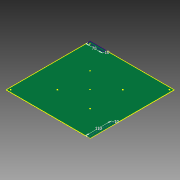
# Autodesk Inventor part: Platine
Saved by Autodesk Inventor 2013 SP1 (Build 170176100, 176)
## iProperties
Created: 2012-12-07
Part Number: Platine
Material: Platinengrün
Document SubType Name: Modeling
Designer: Sebastian
Density: 1 g/cm^3
Author: Sebastian
Autodesk Inventor part; units mm, degrees
ref_plane "YZ Plane" through (0, 0, 0) normal (1, 0, 0) x (0, 1, 0)
ref_plane "XZ Plane" through (0, 0, 0) normal (0, 1, 0) x (-1, 0, 0)
ref_plane "XY Plane" through (0, 0, 0) normal (0, 0, 1) x (1, 0, 0)
sketch "Skizze1" plane through (0, 0, 0) normal (0, 0, 1) x (1, 0, 0)
  line L0 (-180, -180) -> (180, -180)
  line L1 (180, -180) -> (180, 180)
  line L2 (180, 180) -> (-180, 180)
  line L3 (-180, 180) -> (-180, -180)
  line L4 (-180, -180) -> (180, 180) construction
  line L5 (180, -180) -> (-180, 180) construction
  point P0 (0, 0)
  dimension "d0" = 360
  dimension "d1" = 360
  constraints: 12 end point, 2 midpoint, 2 parallel, 1 horizontal, 1 perpendicular
  measures "d0" distance of L2.end L1.end
  measures "d1" distance of L1.end L0.end
extrude "Extrusion1" add sketch "Skizze1" along normal blind 2
hole "Bohrung1" at (-170, -170, 0) direction (0, 0, 1) diameter 3 end through all
pattern_linear "Rechteckige Anordnung1" count 2 spacing 340 along (1, 0, 0) count 2 spacing 340 along (0, 1, 0) of "Bohrung1"
hole "Bohrung2" at (-70, -70, 0) direction (0, 0, 1) diameter 3 end through all
pattern_linear "Rechteckige Anordnung2" count 2 spacing 140 along (1, 0, 0) count 2 spacing 140 along (0, 1, 0) of "Bohrung2"
sketch "Skizze2" plane through (0, 0, 2) normal (0, 0, 1) x (1, 0, 0)
  circle A0 centre (70, 70) radius 1.5 projected
  circle A1 centre (-70, 70) radius 1.5 projected
  circle A2 centre (70, -70) radius 1.5 projected
  circle A3 centre (-70, -70) radius 1.5 projected
  circle A4 centre (170, 170) radius 1.5 projected
  circle A5 centre (-170, 170) radius 1.5 projected
  circle A6 centre (-170, -170) radius 1.5 projected
  line L0 (-180, -180) -> (180, -180) projected
  line L1 (180, -180) -> (180, 180) projected
  line L2 (180, 180) -> (-180, 180) projected
  line L3 (-180, 180) -> (-180, -180) projected
  line L4 (-180, 180) -> (-110, 180)
  line L5 (-110, 180) -> (-110, 170)
  line L6 (-110, 170) -> (-180, 170)
  line L7 (-180, 170) -> (-180, 180)
  line L8 (180, -180) -> (170, -180) construction
  line L9 (170, -180) -> (170, -70) construction
  line L10 (170, -70) -> (180, -70) construction
  line L11 (180, -70) -> (180, -180) construction
  point P0 (0, 0)
  dimension "d34" = 70
  dimension "d35" = 10
  dimension "d38" = 10
  dimension "d39" = 110
  constraints: 16 end point, 4 parallel, 2 horizontal, 2 perpendicular
  measures "d34" distance of L5.end L6.end
  measures "d35" distance of L4.end L5.end
  measures "d38" distance of L9.end L10.end
  measures "d39" distance of L8.end L9.end
